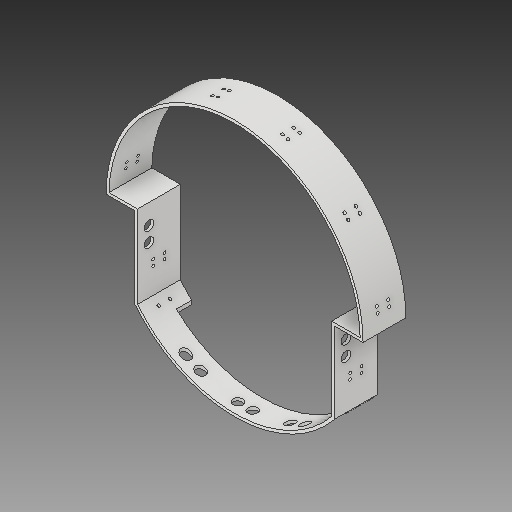
# Autodesk Inventor part: CW000
Saved by Autodesk Inventor 2017 SP1 (Build 210196100, 196)
## iProperties
Created: 2017-05-15
Part Number: CW000
Material: ABS Plastic
Document SubType Name: Modeling
Designer: zallen
Density: 1.06 g/cm^3
Appearance: Smooth - White
Author: zallen
Autodesk Inventor part; units mm, degrees
ref_plane "YZ Plane" through (0, 0, 0) normal (1, 0, 0) x (0, 1, 0)
ref_plane "XZ Plane" through (0, 0, 0) normal (0, 1, 0) x (-1, 0, 0)
ref_plane "XY Plane" through (0, 0, 0) normal (0, 0, 1) x (1, 0, 0)
sketch "Sketch1" plane through (0, 0, 0) normal (0, 0, 1) x (1, 0, 0)
  line L0 (-225, 0) -> (-175, 0) construction
  line L1 (-175, 0) -> (-175, -141.4214) construction
  line L2 (225, 0) -> (175, 0) construction
  line L3 (175, 0) -> (175, -141.4214) construction
  arc A0 (225, 0) -> (-225, 0) centre (0, 0) ccw
  arc A1 (-175, -141.4214) -> (175, -141.4214) centre (0, 0) ccw
  line L4 (-225, 0) -> (-175, 0)
  line L5 (-175, -141.4214) -> (-175, 0)
  line L6 (225, 0) -> (175, 0)
  line L7 (175, -141.4214) -> (175, 0)
  arc A2 (219.9432, 5) -> (-219.9432, 5) centre (0, 0) ccw
  line L8 (219.9432, 5) -> (170, 5)
  line L9 (170, 5) -> (170, -139.6424)
  arc A3 (-170, -139.6424) -> (170, -139.6424) centre (0, 0) ccw
  line L10 (-170, -139.6424) -> (-170, 5)
  line L11 (-170, 5) -> (-219.9432, 5)
  dimension "d1" = 50
  dimension "d2" = 50
  dimension "d3" = 5
  constraints: 24 end point, 8 point on circle, 4 centre point, 4 perpendicular, 3 collinear, 2 horizontal, 5 other
  measures "d1" distance of L0.start L0.end
  measures "d2" distance of L2.start L2.end
  measures "d3" radial gap between concentric circles of A0 A2
extrude "Extrusion1" add sketch "Sketch1" along normal blind 75
sketch "Sketch3" plane through (-175, -141.4214, 0) normal (-1, 0, 0) x (0, 0, 1)
  circle A0 centre (47.5, 46.6338) radius 2.5 projected
  circle A1 centre (47.5, 56.6338) radius 2.5 projected
  circle A2 centre (27.5, 56.6338) radius 2.5 projected
  circle A3 centre (27.5, 46.6338) radius 2.5 projected
  circle A4 centre (47.5, 46.6338) radius 2.5
  circle A5 centre (47.5, 56.6338) radius 2.5
  circle A6 centre (27.5, 56.6338) radius 2.5
  circle A7 centre (27.5, 46.6338) radius 2.5
  point P0 (0, 141.4214)
  constraints: 4 centre point, 4 coincident, 4 concentric
extrude "Extrusion2" cut sketch "Sketch3" against normal through all
ref_plane "Work Plane1" through (261.2863, -247.913, -25.989) normal (0.9880034, 0.154432, 0) x (-0.0534151, 0.3417317, -0.9382783)
sketch "Sketch4" plane through (261.2863, -247.913, -25.989) normal (0.9880034, 0.154432, 0) x (-0.0534151, 0.3417317, -0.9382783)
  circle A0 centre (27.9939, 288.4084) radius 2.5 projected
  circle A1 centre (31.4527, 297.7912) radius 2.5 projected
  circle A2 centre (46.7594, 281.4908) radius 2.5 projected
  circle A3 centre (50.2182, 290.8735) radius 2.5 projected
  circle A4 centre (27.9939, 288.4084) radius 2.5
  circle A5 centre (31.4527, 297.7912) radius 2.5
  circle A6 centre (46.7594, 281.4908) radius 2.5
  circle A7 centre (50.2182, 290.8735) radius 2.5
  point P0 (74.2915, 276.6704)
  constraints: 4 centre point, 4 coincident, 4 concentric
extrude "Extrusion3" cut sketch "Sketch4" along normal through all
ref_plane "Work Plane2" through (669.4541, -423.2188, 1129.6073) normal (0.7480036, 0.6636947, 0) x (-0.5365062, 0.6046584, -0.5886844)
sketch "Sketch5" plane through (669.4541, -423.2188, 1129.6073) normal (0.7480036, 0.6636947, 0) x (-0.5365062, 0.6046584, -0.5886844)
  circle A0 centre (1248.0469, -429.7593) radius 2.5 projected
  circle A1 centre (1256.1306, -423.8725) radius 2.5 projected
  circle A2 centre (1259.8206, -445.9266) radius 2.5 projected
  circle A3 centre (1267.9043, -440.0397) radius 2.5 projected
  circle A4 centre (1248.0469, -429.7593) radius 2.5
  circle A5 centre (1256.1306, -423.8725) radius 2.5
  circle A6 centre (1259.8206, -445.9266) radius 2.5
  circle A7 centre (1267.9043, -440.0397) radius 2.5
  point P0 (1280.0513, -465.2131)
  constraints: 4 centre point, 4 coincident, 4 concentric
extrude "Extrusion4" cut sketch "Sketch5" along normal through all
ref_plane "Work Plane3" through (771.3623, 9.9459, -459.6919) normal (0.2726306, 0.9621188, 0) x (-0.9437667, 0.2674302, 0.1943847)
sketch "Sketch6" plane through (771.3623, 9.9459, -459.6919) normal (0.2726306, 0.9621188, 0) x (-0.9437667, 0.2674302, 0.1943847)
  circle A0 centre (819.012, 354.7554) radius 2.5 projected
  circle A1 centre (828.8212, 352.8116) radius 2.5 projected
  circle A2 centre (815.1243, 335.1369) radius 2.5 projected
  line L0 (814.6833, 307.1895) -> (829.2622, 380.7589) projected
  circle A3 centre (824.9335, 333.1931) radius 2.5 projected
  line L1 (174.5326, 665.6706) -> (209.3762, 727.8919) projected
  circle A4 centre (819.012, 354.7554) radius 2.5
  circle A5 centre (828.8212, 352.8116) radius 2.5
  circle A6 centre (824.9335, 333.1931) radius 2.5
  circle A7 centre (815.1243, 335.1369) radius 2.5
  constraints: 4 centre point, 4 coincident, 4 concentric
extrude "Extrusion5" cut sketch "Sketch6" along normal through all
ref_plane "Work Plane4" through (-2038.7191, -349.1784, 357.9649) normal (-0.2726306, 0.9621188, 0) x (0.3789755, 0.1073883, -0.9191547)
sketch "Sketch7" plane through (-2038.7191, -349.1784, 357.9649) normal (-0.2726306, 0.9621188, 0) x (0.3789755, 0.1073883, -0.9191547)
  circle A0 centre (1093.518, -1763.5263) radius 2.5 projected
  circle A1 centre (1097.457, -1772.7178) radius 2.5 projected
  circle A2 centre (1115.8401, -1764.8399) radius 2.5 projected
  circle A3 centre (1111.9011, -1755.6483) radius 2.5 projected
  circle A4 centre (1093.518, -1763.5263) radius 2.5
  circle A5 centre (1111.9011, -1755.6483) radius 2.5
  circle A6 centre (1115.8401, -1764.8399) radius 2.5
  circle A7 centre (1097.457, -1772.7178) radius 2.5
  point P0 (1139.1474, -1749.412)
  constraints: 4 centre point, 4 coincident, 4 concentric
extrude "Extrusion6" cut sketch "Sketch7" along normal through all
ref_plane "Work Plane5" through (-492.8349, -224.1637, -170.6678) normal (-0.7480036, 0.6636947, 0) x (-0.349588, -0.3939961, 0.8500325)
sketch "Sketch8" plane through (-492.8349, -224.1637, -170.6678) normal (-0.7480036, 0.6636947, 0) x (-0.349588, -0.3939961, 0.8500325)
  circle A0 centre (-77.7927, 539.734) radius 2.5 projected
  circle A1 centre (-72.5254, 531.2336) radius 2.5 projected
  circle A2 centre (-89.5261, 520.699) radius 2.5 projected
  circle A3 centre (-94.7934, 529.1994) radius 2.5 projected
  circle A4 centre (-72.5254, 531.2336) radius 2.5
  circle A5 centre (-89.5261, 520.699) radius 2.5
  circle A6 centre (-94.7934, 529.1994) radius 2.5
  circle A7 centre (-77.7927, 539.734) radius 2.5
  point P0 (-115.5356, 510.4641)
  constraints: 4 centre point, 4 coincident, 4 concentric
extrude "Extrusion7" cut sketch "Sketch8" along normal through all
ref_plane "Work Plane6" through (-128.1534, 603.826, 928.2492) normal (-0.9880034, 0.154432, 0) x (-0.1515994, -0.9698817, 0.190649)
sketch "Sketch9" plane through (-128.1534, 603.826, 928.2492) normal (-0.9880034, 0.154432, 0) x (-0.1515994, -0.9698817, 0.190649)
  circle A0 centre (393.3896, -973.6062) radius 2.5 projected
  circle A1 centre (403.2061, -975.5127) radius 2.5 projected
  circle A2 centre (389.5766, -993.2393) radius 2.5 projected
  circle A3 centre (399.3932, -995.1458) radius 2.5 projected
  circle A4 centre (403.2061, -975.5127) radius 2.5
  circle A5 centre (399.3932, -995.1458) radius 2.5
  circle A6 centre (389.5766, -993.2393) radius 2.5
  circle A7 centre (393.3896, -973.6062) radius 2.5
  point P0 (389.242, -1021.1882)
  constraints: 4 centre point, 4 coincident, 4 concentric
extrude "Extrusion8" cut sketch "Sketch9" along normal through all
ref_plane "Work Plane7" through (-301.178, -7.0894, -544.5578) normal (-0.7135281, -0.7006267, 0) x (-0.69944, 0.7123196, 0.0581765)
sketch "Sketch10" plane through (-301.178, -7.0894, -544.5578) normal (-0.7135281, -0.7006267, 0) x (-0.69944, 0.7123196, 0.0581765)
  circle A0 centre (-166.1706, -602.7459) radius 2.5 projected
  circle A1 centre (-167.3342, -582.7797) radius 2.5 projected
  circle A2 centre (-166.1706, -602.7459) radius 2.5
  circle A3 centre (-167.3342, -582.7797) radius 2.5
  point P0 (-173.9256, -555.6172)
  constraints: 2 centre point, 2 coincident, 2 concentric
extrude "Extrusion9" cut sketch "Sketch10" along normal through all
ref_plane "Work Plane8" through (439.3465, 656.9015, 442.8518) normal (0.9459555, -0.3242964, 0) x (0.0029255, 0.0085334, -0.9999593)
sketch "Sketch11" plane through (439.3465, 656.9015, 442.8518) normal (0.9459555, -0.3242964, 0) x (0.0029255, 0.0085334, -0.9999593)
  circle A0 centre (387.6667, -853.6729) radius 2.5 projected
  circle A1 centre (407.6658, -853.8533) radius 2.5 projected
  circle A2 centre (387.6667, -853.6729) radius 2.5
  circle A3 centre (407.6658, -853.8533) radius 2.5
  point P0 (435.9429, -767.8419)
  constraints: 2 centre point, 2 coincident, 2 concentric
extrude "Extrusion10" cut sketch "Sketch11" along normal through all
ref_plane "Work Plane9" through (-170, -139.6424, 0) normal (0.0051563, 0.9999867, 0) x (0, 0, 1)
sketch "Sketch12" plane through (-170, -139.6424, 0) normal (0.0051563, 0.9999867, 0) x (0, 0, 1)
  line L0 (0, 0) -> (0, 339.9955) projected
  line L1 (0, 20) -> (27, 20)
  line L2 (27, 20) -> (27, 320)
  line L3 (27, 320) -> (0, 320)
  line L4 (0, 320) -> (0, 20)
  point P0 (0, 169.2777)
  dimension "d24" = 27
  dimension "d25" = 20
  dimension "d26" = 300
  constraints: 8 end point, 2 parallel, 1 horizontal, 1 perpendicular, 1 point on line
  measures "d24" distance of L3.end L2.end
  measures "d25" distance from line of L0.start L1
  measures "d26" distance of L1.end L2.end
extrude "Extrusion11" cut sketch "Sketch12" against normal through all
sketch "Sketch13" plane through (175, -141.4214, 0) normal (1, 0, 0) x (0, 0, -1)
  circle A0 centre (-55, 85.4214) radius 8.5
  circle A1 centre (-55, 111.4214) radius 8.5
  line L0 (0, 141.4214) -> (0, 0) projected
  line L1 (0, 141.4214) -> (-75, 141.4214) projected
  dimension "d29" = 17
  dimension "d30" = 17
  dimension "d31" = 26
  dimension "d32" = 55
  dimension "d35" = 30
  constraints: 2 centre point, 1 vertical alignment
  measures "d29" diameter of A0
  measures "d30" diameter of A1
  measures "d31" distance of A1.centre A0.centre
  measures "d32" distance from line of L0 A0.centre
  measures "d35" distance from line of L1 A1.centre
extrude "Extrusion12" cut sketch "Sketch13" against normal through all
sketch "Sketch14" plane through (-170, -139.6424, 0) normal (0.0051563, 0.9999867, 0) x (0, 0, 1)
  circle A0 centre (55, 64.7777) radius 8.5
  circle A1 centre (55, 90.7777) radius 8.5
  circle A2 centre (55, 247.7777) radius 8.5
  circle A3 centre (55, 273.7777) radius 8.5
  circle A4 centre (55, 156.2777) radius 8.5
  circle A5 centre (55, 182.2777) radius 8.5
  point P0 (0, 169.2777)
  dimension "d36" = 17
  dimension "d37" = 17
  dimension "d38" = 26
  dimension "d39" = 17
  dimension "d40" = 17
  dimension "d41" = 26
  dimension "d45" = 17
  dimension "d46" = 17
  dimension "d47" = 26
  dimension "d49" = 13
  dimension "d50" = 65.5
  dimension "d51" = 65.5
  dimension "d52" = 55
  constraints: 6 centre point, 5 vertical alignment
  measures "d36" diameter of A0
  measures "d37" diameter of A1
  measures "d38" distance of A1.centre A0.centre
  measures "d39" diameter of A2
  measures "d40" diameter of A3
  measures "d41" distance of A3.centre A2.centre
  measures "d45" diameter of A4
  measures "d46" diameter of A5
  measures "d47" distance of A5.centre A4.centre
  measures "d49" vertical distance of point (0, 169.278) A4.centre
  measures "d50" distance of A4.centre A1.centre
  measures "d51" distance of A2.centre A5.centre
  measures "d52" horizontal distance of point (0, 169.278) A2.centre
extrude "Extrusion13" cut sketch "Sketch14" against normal through all
body "Solid1"
